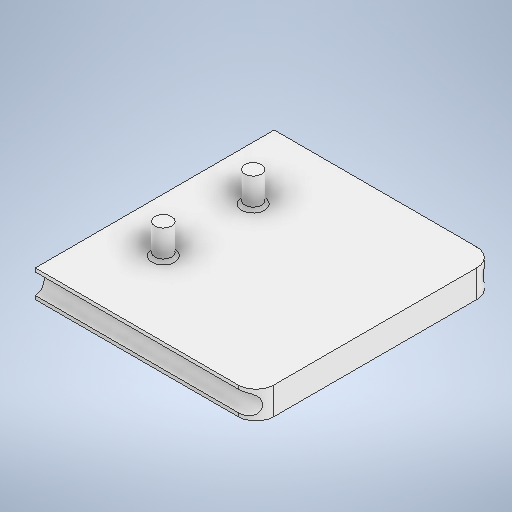
# Autodesk Inventor part: IMU_mount_baseplate
Saved by Autodesk Inventor 2025.2 (Build 292293000, 293)
## iProperties
Created: 2024-11-14
Part Number: IMU_mount_baseplate
Material: Generic
Document SubType Name: Modeling
Designer: matss
Density: 1 g/cm^3
Appearance: Default
Author: matss
Autodesk Inventor part; units mm, degrees
ref_plane "YZ Plane" through (0, 0, 0) normal (1, 0, 0) x (0, 1, 0)
ref_plane "XZ Plane" through (0, 0, 0) normal (0, 1, 0) x (-1, 0, 0)
ref_plane "XY Plane" through (0, 0, 0) normal (0, 0, 1) x (1, 0, 0)
sketch "Sketch1" plane through (0, 0, 0) normal (0, 1, 0) x (-1, 0, 0)
  line L0 (20, 20) -> (-20, 20)
  line L1 (-20, 20) -> (-20, -20)
  line L2 (-20, -20) -> (20, -20)
  line L3 (20, -20) -> (20, 20)
  circle A0 centre (12.5, 12.5) radius 4.25
  circle A1 centre (12.5, -12.5) radius 4.25
  circle A2 centre (-12.5, -12.5) radius 4.25
  circle A3 centre (-12.5, 12.5) radius 4.25
  line L4 (20, 0) -> (-20, 0) construction
  line L5 (0, 20) -> (0, -20) construction
  point P0 (0, 0)
  dimension "d0" = 40
  dimension "d1" = 40
  dimension "d2" = 8.5
  dimension "d3" = 25
  dimension "d4" = 25
  constraints: 12 end point, 4 centre point, 4 midpoint, 3 equal radius, 2 parallel, 1 horizontal, 1 horizontal alignment, 1 perpendicular, 1 vertical alignment, 3 other
  measures "d0" distance of L2.end L0.start
  measures "d1" distance of L0.start L0.end
  measures "d2" diameter of A0
  measures "d3" distance of A1.centre A0.centre
  measures "d4" distance of A3.centre A0.centre
extrude "Extrusion2" add sketch "Sketch1" along normal blind 2
sketch "Sketch2" plane through (0, 0, 0) normal (0, -1, 0) x (1, 0, 0)
  line L0 (20, 20) -> (20, -20) projected
  line L1 (-20, 20) -> (20, 20) projected
  line L2 (-20, -20) -> (-20, 20) projected
  line L3 (20, -20) -> (-20, -20) projected
  point P0 (0, 0)
extrude "Extrusion3" add sketch "Sketch2" along normal blind 0.6
sketch "Sketch3" plane through (0, 2, 0) normal (0, 1, 0) x (1, 0, 0)
  line L0 (-20, 20) -> (-20, -20) projected
  line L1 (-20, -20) -> (20, -20) projected
  line L2 (20, -20) -> (20, 20) projected
  line L3 (20, 20) -> (-20, 20) projected
  point P0 (0, 0)
extrude "Extrusion4" add sketch "Sketch3" along normal blind 2
sketch "Sketch4" plane through (0, 4, 0) normal (0, 1, 0) x (1, 0, 0)
  circle A0 centre (-8, -7.5305) radius 1.4
  circle A1 centre (-8, 7.5305) radius 1.4
  line L0 (-20, -20) -> (-20, 20) projected
  line L1 (-20, 0) -> (20, 0) construction
  line L2 (20, 20) -> (20, -20) projected
  point P0 (0, 0)
  dimension "d13" = 15.061
  dimension "d14" = 2.8
  dimension "d15" = 12
  constraints: 2 centre point, 2 end point, 2 midpoint, 1 equal radius, 1 other
  measures "d13" distance of A1.centre A0.centre
  measures "d14" diameter of A0
  measures "d15" distance from line of L0 A1.centre
extrude "Extrusion5" add sketch "Sketch4" along normal blind 5
chamfer "Chamfer1" distance 0.5 angle 45 2 edges at (-9.4, 4, 7.5305) (-9.4, 4, -7.5305)
fillet "Fillet1" radius 3 4 edges at (-20, 1.7, 20) (-20, 1.7, -20) (20, 1.7, 20) (20, 1.7, -20)
ref_plane "Arbeitsebene1" through (-17, 4, 20) normal (1, 0, 0) x (0, -1, 0)
sketch "Skizze5" plane through (-17, 4, 20) normal (1, 0, 0) x (0, -1, 0)
  line L0 (0, 0) -> (4.6, 0) construction
  line L1 (0, 0) -> (0, 3) construction
  line L2 (0.7, 0) -> (4, 0) construction
  line L3 (6.1491, 20) -> (-1.642, 20) construction
  line L4 (0, 40) -> (4.6, 40) construction
  line L5 (0.7, 40) -> (4, 40) construction
  line L6 (2.3, 0) -> (2.3, 4.6722) construction
  ellipse E0 centre (2.3, 0) end of major axis (4, 0) minor radius 1.5
  line L7 (0.6, 0) -> (4, 0)
  line L8 (0, 40) -> (4.6, 40) construction
  line L9 (0.7, 40) -> (4, 40) construction
  ellipse E1 centre (2.3, 40) end of major axis (4, 40) minor radius 1.5
  line L10 (0.6, 40) -> (4, 40)
  point P0 (4, 20)
  point P1 (2.3, 1.5)
  dimension "d22" = 2.3
  dimension "d23" = 1.7
  dimension "d28" = 1.5
  constraints: 18 end point, 9 point on line, 6 symmetric about line, 3 horizontal, 2 collinear, 2 midpoint, 1 coincident, 1 vertical, 9 other
  measures "d22" distance from line of L1 L6.start
  measures "d23" distance of L6.start L2.end
  measures "d28" distance of point (2.3, 0) point (2.3, 1.5)
extrude "Extrusion7" cut sketch "Skizze5" along normal blind 37 and the other way blind 5 contours L7 E0 | E1 L10 picked at (2.3489, 0.4981) picked at (2.2511, 39.5019)
body "Solid2"
